Autodesk Fusion 360 part; units mm, degrees
(part 3 of 4)
  arc A110 (-253.4839, 110.4829) -> (-253.0782, 110.7207) centre (-253.4447, 110.881) ccw
  arc A111 (-251.1958, 114.9274) -> (-251.2888, 115.3883) centre (-251.5595, 115.0938) ccw
  arc A112 (-273.2935, 80.8439) -> (-274.4157, 76.9484) centre (0, 0) ccw
  spline S113 degree 3 poles (-273.2935, 80.8439) (-270.7574, 81.1159) (-268.4259, 81.2764) (-266.3051, 81.3548) knots 0 0 0 0 1 1 1 1
  spline S114 degree 3 poles (-270.6648, 56.5783) (-271.2365, 56.9046) (-271.8248, 57.2492) (-272.4294, 57.6132) knots 0 0 0 0 1 1 1 1
  arc A113 (-251.1958, 114.9274) -> (-253.0782, 110.7207) centre (0, 0) ccw
  arc A114 (-266.8977, 71.2268) -> (-267.0666, 71.6656) centre (-267.2842, 71.3299) ccw
  spline S115 degree 3 poles (-255.5218, 110.66) (-254.8182, 110.607) (-254.1389, 110.5476) (-253.4839, 110.4829) knots 0 0 0 0 1 1 1 1
  spline S116 degree 3 poles (-266.3051, 81.3548) (-265.6, 81.381) (-264.9183, 81.398) (-264.2602, 81.407) knots 0 0 0 0 1 1 1 1
  arc A115 (-246.8902, 124.5221) -> (-246.4719, 124.7367) centre (-246.8288, 124.9173) ccw
  arc A116 (-244.3566, 128.8313) -> (-246.4719, 124.7367) centre (0, 0) ccw
  arc A117 (-248.452, 139.6305) -> (-250.4129, 136.0824) centre (0, 0) ccw
  spline S117 degree 3 poles (-267.0666, 71.6656) (-267.6191, 72.0234) (-268.1872, 72.4005) (-268.7704, 72.7978) knots 0 0 0 0 1 1 1 1
  arc A118 (-274.1626, 35.9916) -> (-273.8386, 36.3324) centre (-274.2352, 36.385) ccw
  spline S118 degree 3 poles (-275.2312, 42.2473) (-277.1078, 43.2382) (-279.1389, 44.3943) (-281.3058, 45.7398) knots 0 0 0 0 1 1 1 1
  spline S119 degree 3 poles (-248.9151, 124.8131) (-248.2155, 124.7208) (-247.5406, 124.6234) (-246.8902, 124.5221) knots 0 0 0 0 1 1 1 1
  arc A119 (-273.1944, 40.8958) -> (-273.4114, 41.313) centre (-273.59, 40.9551) ccw
  spline S120 degree 3 poles (-245.8327, 130.7796) (-247.2768, 132.3347) (-248.812, 134.0968) (-250.4129, 136.0824) knots 0 0 0 0 1 1 1 1
  spline S121 degree 3 poles (-261.3246, 96.1587) (-260.6191, 96.1452) (-259.9375, 96.124) (-259.2799, 96.0962) knots 0 0 0 0 1 1 1 1
  spline S122 degree 3 poles (-251.2888, 115.3883) (-251.7735, 115.8336) (-252.2705, 116.3006) (-252.7789, 116.7899) knots 0 0 0 0 1 1 1 1
  arc A120 (-236.7485, 142.3298) -> (-239.0901, 138.3603) centre (0, 0) ccw
  arc A121 (-273.1944, 40.8958) -> (-273.8386, 36.3324) centre (0, 0) ccw
  arc A122 (-270.4716, 56.1496) -> (-270.6648, 56.5783) centre (-270.8632, 56.2309) ccw
  spline S123 degree 3 poles (-268.3306, 96.0404) (-265.7832, 96.1698) (-263.4464, 96.1992) (-261.3246, 96.1587) knots 0 0 0 0 1 1 1 1
  arc A123 (-268.409, 66.4618) -> (-268.0489, 66.7641) centre (-268.437, 66.8608) ccw
  spline S124 degree 3 poles (-257.3634, 101.1169) (-257.8723, 101.5344) (-258.3946, 101.9727) (-258.9296, 102.4328) knots 0 0 0 0 1 1 1 1
  spline S125 degree 3 poles (-268.7704, 72.7978) (-270.5243, 73.9925) (-272.4131, 75.3688) (-274.4157, 76.9484) knots 0 0 0 0 1 1 1 1
  arc A124 (-262.4841, 86.0798) -> (-262.6282, 86.5274) centre (-262.8642, 86.2044) ccw
  spline S126 degree 3 poles (-255.8902, 125.48) (-253.3445, 125.3234) (-251.019, 125.091) (-248.9151, 124.8131) knots 0 0 0 0 1 1 1 1
  arc A125 (-280.6267, 49.7364) -> (-281.3058, 45.7398) centre (0, 0) ccw
  arc A126 (-270.4716, 56.1496) -> (-271.3707, 51.6295) centre (0, 0) ccw
  arc A127 (-255.8902, 125.48) -> (-257.6492, 121.8275) centre (0, 0) ccw
  spline S127 degree 3 poles (-272.4294, 57.6132) (-274.2475, 58.7077) (-276.2105, 59.9759) (-278.2986, 61.4407) knots 0 0 0 0 1 1 1 1
  arc A128 (-262.4841, 86.0798) -> (-263.8837, 81.6887) centre (0, 0) ccw
  spline S128 degree 3 poles (-280.6267, 49.7364) (-278.137, 50.2907) (-275.8381, 50.7111) (-273.7395, 51.0266) knots 0 0 0 0 1 1 1 1
  arc A129 (-277.3965, 65.393) -> (-278.2986, 61.4407) centre (0, 0) ccw
  arc A130 (-264.2602, 81.407) -> (-263.8837, 81.6887) centre (-264.2658, 81.807) ccw
  arc A131 (-257.2447, 100.662) -> (-257.3634, 101.1169) centre (-257.6171, 100.8077) ccw
  arc A132 (-268.3306, 96.0404) -> (-269.6695, 92.214) centre (0, 0) ccw
  arc A133 (-262.5234, 110.9347) -> (-264.0748, 107.1894) centre (0, 0) ccw
  spline S129 degree 3 poles (-273.4114, 41.313) (-274.0004, 41.6067) (-274.6072, 41.9178) (-275.2312, 42.2473) knots 0 0 0 0 1 1 1 1
  spline S130 degree 3 poles (-270.4478, 66.295) (-269.7452, 66.3606) (-269.0656, 66.4158) (-268.409, 66.4618) knots 0 0 0 0 1 1 1 1
  spline S131 degree 3 poles (-252.7789, 116.7899) (-254.3079, 118.2616) (-255.9395, 119.9348) (-257.6492, 121.8275) knots 0 0 0 0 1 1 1 1
  spline S132 degree 3 poles (-264.2658, 87.7533) (-265.9499, 89.0445) (-267.7586, 90.5246) (-269.6695, 92.214) knots 0 0 0 0 1 1 1 1
  arc A134 (-271.7132, 51.3074) -> (-271.3707, 51.6295) centre (-271.7636, 51.7042) ccw
  arc A135 (-257.2447, 100.662) -> (-258.8882, 96.3563) centre (0, 0) ccw
  arc A136 (-244.3566, 128.8313) -> (-244.4236, 129.2967) centre (-244.7104, 129.0178) ccw
  spline S133 degree 3 poles (-244.4236, 129.2967) (-244.8826, 129.7685) (-245.3526, 130.2625) (-245.8327, 130.7796) knots 0 0 0 0 1 1 1 1
  spline S134 degree 3 poles (-262.6282, 86.5274) (-263.1597, 86.9156) (-263.7058, 87.324) (-264.2658, 87.7533) knots 0 0 0 0 1 1 1 1
  spline S135 degree 3 poles (-276.1699, 35.5976) (-275.4792, 35.7415) (-274.81, 35.8724) (-274.1626, 35.9916) knots 0 0 0 0 1 1 1 1
  spline S136 degree 3 poles (-273.7395, 51.0266) (-273.0417, 51.1315) (-272.3662, 51.2247) (-271.7132, 51.3074) knots 0 0 0 0 1 1 1 1
  spline S137 degree 3 poles (-258.9296, 102.4328) (-260.5388, 103.8164) (-262.2616, 105.3955) (-264.0748, 107.1894) knots 0 0 0 0 1 1 1 1
  arc A137 (-259.2799, 96.0962) -> (-258.8882, 96.3563) centre (-259.2631, 96.4958) ccw
  arc A138 (-236.7485, 142.3298) -> (-236.7894, 142.7982) centre (-237.0914, 142.5359) ccw
  spline S138 degree 3 poles (-224.4912, 164.7445) (-223.817, 164.5362) (-223.1679, 164.3272) (-222.5437, 164.1184) knots 0 0 0 0 1 1 1 1
  arc A139 (-209.5624, 179.9757) -> (-212.5358, 176.4544) centre (0, 0) ccw
  arc A140 (-211.152, 191.4154) -> (-213.8534, 188.3926) centre (0, 0) ccw
  spline S139 degree 3 poles (-248.452, 139.6305) (-245.919, 139.3314) (-243.6102, 138.969) (-241.5251, 138.5736) knots 0 0 0 0 1 1 1 1
  arc A141 (-231.3958, 151.382) -> (-230.9561, 151.5485) centre (-231.2905, 151.7679) ccw
  spline S140 degree 3 poles (-241.5251, 138.5736) (-240.8319, 138.4421) (-240.1635, 138.307) (-239.5198, 138.1694) knots 0 0 0 0 1 1 1 1
  spline S141 degree 3 poles (-219.3122, 168.4123) (-219.6856, 168.9543) (-220.0662, 169.5201) (-220.453, 170.1103) knots 0 0 0 0 1 1 1 1
  spline S142 degree 3 poles (-231.2561, 166.5703) (-228.7725, 165.9895) (-226.5188, 165.3708) (-224.4912, 164.7445) knots 0 0 0 0 1 1 1 1
  arc A142 (-222.5437, 164.1184) -> (-222.0953, 164.2599) centre (-222.4169, 164.4977) ccw
  arc A143 (-219.324, 167.9423) -> (-222.0953, 164.2599) centre (0, 0) ccw
  arc A144 (-209.5624, 179.9757) -> (-209.5242, 180.4443) centre (-209.8658, 180.2363) ccw
  spline S143 degree 3 poles (-211.152, 191.4154) (-208.7491, 190.5602) (-206.5789, 189.6931) (-204.6341, 188.8436) knots 0 0 0 0 1 1 1 1
  spline S144 degree 3 poles (-204.6341, 188.8436) (-203.9875, 188.5612) (-203.3659, 188.2808) (-202.769, 188.0034) knots 0 0 0 0 1 1 1 1
  arc A145 (-200.0871, 202.9537) -> (-202.9537, 200.0871) centre (0, 0) ccw
  spline S145 degree 3 poles (-228.4101, 155.8505) (-228.8134, 156.3707) (-229.2251, 156.9142) (-229.6443, 157.4818) knots 0 0 0 0 1 1 1 1
  spline S146 degree 3 poles (-199.077, 191.9086) (-199.3874, 192.489) (-199.7023, 193.0938) (-200.0205, 193.7236) knots 0 0 0 0 1 1 1 1
  arc A146 (-219.324, 167.9423) -> (-219.3122, 168.4123) centre (-219.6416, 168.1855) ccw
  spline S147 degree 3 poles (-200.0205, 193.7236) (-200.9776, 195.6177) (-201.965, 197.7359) (-202.9537, 200.0871) knots 0 0 0 0 1 1 1 1
  spline S148 degree 3 poles (-236.7894, 142.7982) (-237.2212, 143.295) (-237.6627, 143.8146) (-238.1131, 144.3578) knots 0 0 0 0 1 1 1 1
  spline S149 degree 3 poles (-238.1131, 144.3578) (-239.4677, 145.9914) (-240.9017, 147.8368) (-242.3888, 149.9091) knots 0 0 0 0 1 1 1 1
  spline S150 degree 3 poles (-233.3753, 151.898) (-232.6905, 151.7279) (-232.0307, 151.5555) (-231.3958, 151.382) knots 0 0 0 0 1 1 1 1
  spline S151 degree 3 poles (-214.9007, 177.0726) (-214.2393, 176.8269) (-213.6029, 176.5818) (-212.9914, 176.3383) knots 0 0 0 0 1 1 1 1
  arc A147 (-199.1414, 191.4428) -> (-199.077, 191.9086) centre (-199.4298, 191.72) ccw
  spline S152 degree 3 poles (-193.7236, 200.0205) (-193.0938, 199.7023) (-192.489, 199.3874) (-191.9086, 199.077) knots 0 0 0 0 1 1 1 1
  arc A148 (-228.3956, 155.3805) -> (-230.9561, 151.5485) centre (0, 0) ccw
  arc A149 (-221.5526, 179.2749) -> (-224.0802, 176.1054) centre (0, 0) ccw
  arc A150 (-199.1414, 191.4428) -> (-202.3076, 188.0938) centre (0, 0) ccw
  spline S153 degree 3 poles (-220.453, 170.1103) (-221.6162, 171.8853) (-222.8345, 173.8797) (-224.0802, 176.1054) knots 0 0 0 0 1 1 1 1
  arc A151 (-228.3956, 155.3805) -> (-228.4101, 155.8505) centre (-228.7263, 155.6055) ccw
  arc A152 (-212.9914, 176.3383) -> (-212.5358, 176.4544) centre (-212.8436, 176.71) ccw
  arc A153 (-202.769, 188.0034) -> (-202.3076, 188.0938) centre (-202.6005, 188.3662) ccw
  arc A154 (-188.0938, 202.3076) -> (-191.4428, 199.1414) centre (0, 0) ccw
  arc A155 (-188.0938, 202.3076) -> (-188.0034, 202.769) centre (-188.3662, 202.6005) ccw
  arc A156 (-239.5198, 138.1694) -> (-239.0901, 138.3603) centre (-239.4363, 138.5606) ccw
  arc A157 (-240.232, 153.3416) -> (-242.3888, 149.9091) centre (0, 0) ccw
  spline S154 degree 3 poles (-200.0871, 202.9537) (-197.7359, 201.965) (-195.6177, 200.9776) (-193.7236, 200.0205) knots 0 0 0 0 1 1 1 1
  spline S155 degree 3 poles (-209.5242, 180.4443) (-209.8667, 181.0064) (-210.2149, 181.5927) (-210.568, 182.2036) knots 0 0 0 0 1 1 1 1
  spline S156 degree 3 poles (-210.568, 182.2036) (-211.6298, 184.041) (-212.7344, 186.1006) (-213.8534, 188.3926) knots 0 0 0 0 1 1 1 1
  spline S157 degree 3 poles (-240.232, 153.3416) (-237.7197, 152.901) (-235.4349, 152.4097) (-233.3753, 151.898) knots 0 0 0 0 1 1 1 1
  spline S158 degree 3 poles (-229.6443, 157.4818) (-230.9052, 159.1888) (-232.2335, 161.1117) (-233.602, 163.2641) knots 0 0 0 0 1 1 1 1
  arc A158 (-231.2561, 166.5703) -> (-233.602, 163.2641) centre (0, 0) ccw
  spline S159 degree 3 poles (-221.5526, 179.2749) (-219.1055, 178.5557) (-216.89, 177.8117) (-214.9007, 177.0726) knots 0 0 0 0 1 1 1 1
  spline S160 degree 3 poles (-188.0034, 202.769) (-188.2808, 203.3659) (-188.5612, 203.9875) (-188.8436, 204.6341) knots 0 0 0 0 1 1 1 1
  arc A159 (-164.2599, 222.0953) -> (-167.9423, 219.324) centre (0, 0) ccw
  arc A160 (-155.3805, -228.3956) -> (-155.8505, -228.4101) centre (-155.6055, -228.7263) ccw
  arc A161 (-176.4544, 212.5358) -> (-179.9757, 209.5624) centre (0, 0) ccw
  arc A162 (-168.4123, 219.3122) -> (-167.9423, 219.324) centre (-168.1855, 219.6416) ccw
  spline S161 degree 3 poles (-177.0726, 214.9007) (-177.8117, 216.89) (-178.5557, 219.1055) (-179.2749, 221.5526) knots 0 0 0 0 1 1 1 1
  arc A163 (-151.5485, 230.9561) -> (-155.3805, 228.3956) centre (0, 0) ccw
  arc A164 (-155.3805, -228.3956) -> (-151.5485, -230.9561) centre (0, 0) ccw
  spline S162 degree 3 poles (-157.4818, -229.6443) (-159.1888, -230.9052) (-161.1117, -232.2335) (-163.2641, -233.602) knots 0 0 0 0 1 1 1 1
  arc A165 (-167.9423, -219.324) -> (-168.4123, -219.3122) centre (-168.1855, -219.6416) ccw
  spline S163 degree 3 poles (-168.4123, -219.3122) (-168.9543, -219.6856) (-169.5201, -220.0662) (-170.1103, -220.453) knots 0 0 0 0 1 1 1 1
  spline S164 degree 3 poles (-179.2749, -221.5526) (-178.5557, -219.1055) (-177.8117, -216.89) (-177.0726, -214.9007) knots 0 0 0 0 1 1 1 1
  spline S165 degree 3 poles (-188.8436, 204.6341) (-189.6931, 206.5789) (-190.5602, 208.7491) (-191.4154, 211.152) knots 0 0 0 0 1 1 1 1
  arc A166 (-164.2599, 222.0953) -> (-164.1184, 222.5437) centre (-164.4977, 222.4169) ccw
  spline S166 degree 3 poles (-153.3416, -240.232) (-152.901, -237.7197) (-152.4097, -235.4349) (-151.898, -233.3753) knots 0 0 0 0 1 1 1 1
  spline S167 degree 3 poles (-180.4443, -209.5242) (-181.0064, -209.8667) (-181.5927, -210.2149) (-182.2036, -210.568) knots 0 0 0 0 1 1 1 1
  arc A167 (-176.1054, 224.0802) -> (-179.2749, 221.5526) centre (0, 0) ccw
  spline S168 degree 3 poles (-151.382, 231.3958) (-151.5555, 232.0307) (-151.7279, 232.6905) (-151.898, 233.3753) knots 0 0 0 0 1 1 1 1
  arc A168 (-151.382, -231.3958) -> (-151.5485, -230.9561) centre (-151.7679, -231.2905) ccw
  arc A169 (-179.9757, -209.5624) -> (-176.4544, -212.5358) centre (0, 0) ccw
  arc A170 (-179.9757, -209.5624) -> (-180.4443, -209.5242) centre (-180.2363, -209.8658) ccw
  spline S169 degree 3 poles (-176.1054, 224.0802) (-173.8797, 222.8345) (-171.8853, 221.6162) (-170.1103, 220.453) knots 0 0 0 0 1 1 1 1
  arc A171 (-191.9086, 199.077) -> (-191.4428, 199.1414) centre (-191.72, 199.4298) ccw
  spline S170 degree 3 poles (-164.1184, 222.5437) (-164.3272, 223.1679) (-164.5362, 223.817) (-164.7445, 224.4912) knots 0 0 0 0 1 1 1 1
  spline S171 degree 3 poles (-170.1103, 220.453) (-169.5201, 220.0662) (-168.9543, 219.6856) (-168.4123, 219.3122) knots 0 0 0 0 1 1 1 1
  spline S172 degree 3 poles (-151.898, 233.3753) (-152.4097, 235.4349) (-152.901, 237.7197) (-153.3416, 240.232) knots 0 0 0 0 1 1 1 1
  arc A172 (-155.8505, 228.4101) -> (-155.3805, 228.3956) centre (-155.6055, 228.7263) ccw
  arc A173 (-188.3926, 213.8534) -> (-191.4154, 211.152) centre (0, 0) ccw
  spline S173 degree 3 poles (-188.3926, 213.8534) (-186.1006, 212.7344) (-184.041, 211.6298) (-182.2036, 210.568) knots 0 0 0 0 1 1 1 1
  arc A174 (-149.9091, 242.3888) -> (-153.3416, 240.232) centre (0, 0) ccw
  spline S174 degree 3 poles (-151.898, -233.3753) (-151.7279, -232.6905) (-151.5555, -232.0307) (-151.382, -231.3958) knots 0 0 0 0 1 1 1 1
  spline S175 degree 3 poles (-164.7445, -224.4912) (-164.5362, -223.817) (-164.3272, -223.1679) (-164.1184, -222.5437) knots 0 0 0 0 1 1 1 1
  spline S176 degree 3 poles (-155.8505, -228.4101) (-156.3707, -228.8134) (-156.9142, -229.2251) (-157.4818, -229.6443) knots 0 0 0 0 1 1 1 1
  spline S177 degree 3 poles (-191.4154, -211.152) (-190.5602, -208.7491) (-189.6931, -206.5789) (-188.8436, -204.6341) knots 0 0 0 0 1 1 1 1
  spline S178 degree 3 poles (-177.0726, -214.9007) (-176.8269, -214.2393) (-176.5818, -213.6029) (-176.3383, -212.9914) knots 0 0 0 0 1 1 1 1
  arc A175 (-180.4443, 209.5242) -> (-179.9757, 209.5624) centre (-180.2363, 209.8658) ccw
  spline S179 degree 3 poles (-182.2036, -210.568) (-184.041, -211.6298) (-186.1006, -212.7344) (-188.3926, -213.8534) knots 0 0 0 0 1 1 1 1
  spline S180 degree 3 poles (-182.2036, 210.568) (-181.5927, 210.2149) (-181.0064, 209.8667) (-180.4443, 209.5242) knots 0 0 0 0 1 1 1 1
  arc A176 (-164.1184, -222.5437) -> (-164.2599, -222.0953) centre (-164.4977, -222.4169) ccw
  spline S181 degree 3 poles (-176.3383, 212.9914) (-176.5818, 213.6029) (-176.8269, 214.2393) (-177.0726, 214.9007) knots 0 0 0 0 1 1 1 1
  arc A177 (-151.5485, 230.9561) -> (-151.382, 231.3958) centre (-151.7679, 231.2905) ccw
  arc A178 (-166.5703, -231.2561) -> (-163.2641, -233.602) centre (0, 0) ccw
  spline S182 degree 3 poles (-170.1103, -220.453) (-171.8853, -221.6162) (-173.8797, -222.8345) (-176.1054, -224.0802) knots 0 0 0 0 1 1 1 1
  arc A179 (-179.2749, -221.5526) -> (-176.1054, -224.0802) centre (0, 0) ccw
  arc A180 (-176.3383, -212.9914) -> (-176.4544, -212.5358) centre (-176.71, -212.8436) ccw
  arc A181 (-163.2641, 233.602) -> (-166.5703, 231.2561) centre (0, 0) ccw
  arc A182 (-191.4154, -211.152) -> (-188.3926, -213.8534) centre (0, 0) ccw
  spline S183 degree 3 poles (-188.8436, -204.6341) (-188.5612, -203.9875) (-188.2808, -203.3659) (-188.0034, -202.769) knots 0 0 0 0 1 1 1 1
  spline S184 degree 3 poles (-166.5703, -231.2561) (-165.9895, -228.7725) (-165.3708, -226.5188) (-164.7445, -224.4912) knots 0 0 0 0 1 1 1 1
  arc A183 (-191.4428, -199.1414) -> (-188.0938, -202.3076) centre (0, 0) ccw
  arc A184 (-191.4428, -199.1414) -> (-191.9086, -199.077) centre (-191.72, -199.4298) ccw
  spline S185 degree 3 poles (-191.9086, -199.077) (-192.489, -199.3874) (-193.0938, -199.7023) (-193.7236, -200.0205) knots 0 0 0 0 1 1 1 1
  spline S186 degree 3 poles (-193.7236, -200.0205) (-195.6177, -200.9776) (-197.7359, -201.965) (-200.0871, -202.9537) knots 0 0 0 0 1 1 1 1
  spline S187 degree 3 poles (-157.4818, 229.6443) (-156.9142, 229.2251) (-156.3707, 228.8134) (-155.8505, 228.4101) knots 0 0 0 0 1 1 1 1
  arc A185 (-167.9423, -219.324) -> (-164.2599, -222.0953) centre (0, 0) ccw
  arc A186 (-188.0034, -202.769) -> (-188.0938, -202.3076) centre (-188.3662, -202.6005) ccw
  arc A187 (-202.9537, -200.0871) -> (-200.0871, -202.9537) centre (0, 0) ccw
  arc A188 (-176.4544, 212.5358) -> (-176.3383, 212.9914) centre (-176.71, 212.8436) ccw
  spline S188 degree 3 poles (-164.7445, 224.4912) (-165.3708, 226.5188) (-165.9895, 228.7725) (-166.5703, 231.2561) knots 0 0 0 0 1 1 1 1
  spline S189 degree 3 poles (-163.2641, 233.602) (-161.1117, 232.2335) (-159.1888, 230.9052) (-157.4818, 229.6443) knots 0 0 0 0 1 1 1 1
  spline S190 degree 3 poles (-224.4912, -164.7445) (-226.5188, -165.3708) (-228.7725, -165.9895) (-231.2561, -166.5703) knots 0 0 0 0 1 1 1 1
  spline S191 degree 3 poles (-204.6341, -188.8436) (-206.5789, -189.6931) (-208.7491, -190.5602) (-211.152, -191.4154) knots 0 0 0 0 1 1 1 1
  spline S192 degree 3 poles (-214.9007, -177.0726) (-216.89, -177.8117) (-219.1055, -178.5557) (-221.5526, -179.2749) knots 0 0 0 0 1 1 1 1
  arc A189 (-239.0901, -138.3603) -> (-236.7485, -142.3298) centre (0, 0) ccw
  arc A190 (-242.3888, -149.9091) -> (-240.232, -153.3416) centre (0, 0) ccw
  arc A191 (-222.0953, -164.2599) -> (-219.324, -167.9423) centre (0, 0) ccw
  arc A192 (-222.0953, -164.2599) -> (-222.5437, -164.1184) centre (-222.4169, -164.4977) ccw
  arc A193 (-199.077, -191.9086) -> (-199.1414, -191.4428) centre (-199.4298, -191.72) ccw
  arc A194 (-212.5358, -176.4544) -> (-209.5624, -179.9757) centre (0, 0) ccw
  arc A195 (-212.5358, -176.4544) -> (-212.9914, -176.3383) centre (-212.8436, -176.71) ccw
  spline S193 degree 3 poles (-212.9914, -176.3383) (-213.6029, -176.5818) (-214.2393, -176.8269) (-214.9007, -177.0726) knots 0 0 0 0 1 1 1 1
  arc A196 (-236.7894, -142.7982) -> (-236.7485, -142.3298) centre (-237.0914, -142.5359) ccw
  arc A197 (-246.4719, -124.7367) -> (-244.3566, -128.8313) centre (0, 0) ccw
  spline S194 degree 3 poles (-224.0802, -176.1054) (-222.8345, -173.8797) (-221.6162, -171.8853) (-220.453, -170.1103) knots 0 0 0 0 1 1 1 1
  spline S195 degree 3 poles (-231.3958, -151.382) (-232.0307, -151.5555) (-232.6905, -151.7279) (-233.3753, -151.898) knots 0 0 0 0 1 1 1 1
  spline S196 degree 3 poles (-238.1131, -144.3578) (-237.6627, -143.8146) (-237.2212, -143.295) (-236.7894, -142.7982) knots 0 0 0 0 1 1 1 1
  arc A198 (-219.3122, -168.4123) -> (-219.324, -167.9423) centre (-219.6416, -168.1855) ccw
  spline S197 degree 3 poles (-220.453, -170.1103) (-220.0662, -169.5201) (-219.6856, -168.9543) (-219.3122, -168.4123) knots 0 0 0 0 1 1 1 1
  spline S198 degree 3 poles (-200.0205, -193.7236) (-199.7023, -193.0938) (-199.3874, -192.489) (-199.077, -191.9086) knots 0 0 0 0 1 1 1 1
  arc A199 (-233.602, -163.2641) -> (-231.2561, -166.5703) centre (0, 0) ccw
  spline S199 degree 3 poles (-222.5437, -164.1184) (-223.1679, -164.3272) (-223.817, -164.5362) (-224.4912, -164.7445) knots 0 0 0 0 1 1 1 1
  arc A200 (-209.5242, -180.4443) -> (-209.5624, -179.9757) centre (-209.8658, -180.2363) ccw
  arc A201 (-228.4101, -155.8505) -> (-228.3956, -155.3805) centre (-228.7263, -155.6055) ccw
  spline S200 degree 3 poles (-229.6443, -157.4818) (-229.2251, -156.9142) (-228.8134, -156.3707) (-228.4101, -155.8505) knots 0 0 0 0 1 1 1 1
  arc A202 (-213.8534, -188.3926) -> (-211.152, -191.4154) centre (0, 0) ccw
  arc A203 (-239.0901, -138.3603) -> (-239.5198, -138.1694) centre (-239.4363, -138.5606) ccw
  spline S201 degree 3 poles (-241.5251, -138.5736) (-243.6102, -138.969) (-245.919, -139.3314) (-248.452, -139.6305) knots 0 0 0 0 1 1 1 1
  spline S202 degree 3 poles (-245.8327, -130.7796) (-245.3526, -130.2625) (-244.8826, -129.7685) (-244.4236, -129.2967) knots 0 0 0 0 1 1 1 1
  arc A204 (-246.4719, -124.7367) -> (-246.8902, -124.5221) centre (-246.8288, -124.9173) ccw
  arc A205 (-202.3076, -188.0938) -> (-199.1414, -191.4428) centre (0, 0) ccw
  arc A206 (-202.3076, -188.0938) -> (-202.769, -188.0034) centre (-202.6005, -188.3662) ccw
  spline S203 degree 3 poles (-202.9537, -200.0871) (-201.965, -197.7359) (-200.9776, -195.6177) (-200.0205, -193.7236) knots 0 0 0 0 1 1 1 1
  spline S204 degree 3 poles (-233.602, -163.2641) (-232.2335, -161.1117) (-230.9052, -159.1888) (-229.6443, -157.4818) knots 0 0 0 0 1 1 1 1
  arc A207 (-230.9561, -151.5485) -> (-228.3956, -155.3805) centre (0, 0) ccw
  arc A208 (-230.9561, -151.5485) -> (-231.3958, -151.382) centre (-231.2905, -151.7679) ccw
  spline S205 degree 3 poles (-239.5198, -138.1694) (-240.1635, -138.307) (-240.8319, -138.4421) (-241.5251, -138.5736) knots 0 0 0 0 1 1 1 1
  arc A209 (-244.4236, -129.2967) -> (-244.3566, -128.8313) centre (-244.7104, -129.0178) ccw
  spline S206 degree 3 poles (-246.8902, -124.5221) (-247.5406, -124.6234) (-248.2155, -124.7208) (-248.9151, -124.8131) knots 0 0 0 0 1 1 1 1
  spline S207 degree 3 poles (-202.769, -188.0034) (-203.3659, -188.2808) (-203.9875, -188.5612) (-204.6341, -188.8436) knots 0 0 0 0 1 1 1 1
  spline S208 degree 3 poles (-248.9151, -124.8131) (-251.019, -125.091) (-253.3445, -125.3234) (-255.8902, -125.48) knots 0 0 0 0 1 1 1 1
  arc A210 (-224.0802, -176.1054) -> (-221.5526, -179.2749) centre (0, 0) ccw
  arc A211 (-257.6492, -121.8275) -> (-255.8902, -125.48) centre (0, 0) ccw
  spline S209 degree 3 poles (-213.8534, -188.3926) (-212.7344, -186.1006) (-211.6298, -184.041) (-210.568, -182.2036) knots 0 0 0 0 1 1 1 1
  spline S210 degree 3 poles (-210.568, -182.2036) (-210.2149, -181.5927) (-209.8667, -181.0064) (-209.5242, -180.4443) knots 0 0 0 0 1 1 1 1
  spline S211 degree 3 poles (-250.4129, -136.0824) (-248.812, -134.0968) (-247.2768, -132.3347) (-245.8327, -130.7796) knots 0 0 0 0 1 1 1 1
  spline S212 degree 3 poles (-242.3888, -149.9091) (-240.9017, -147.8368) (-239.4677, -145.9914) (-238.1131, -144.3578) knots 0 0 0 0 1 1 1 1
  arc A212 (-250.4129, -136.0824) -> (-248.452, -139.6305) centre (0, 0) ccw
  spline S213 degree 3 poles (-233.3753, -151.898) (-235.4349, -152.4097) (-237.7197, -152.901) (-240.232, -153.3416) knots 0 0 0 0 1 1 1 1
  spline S214 degree 3 poles (-266.3051, -81.3548) (-268.4259, -81.2764) (-270.7574, -81.1159) (-273.2935, -80.8439) knots 0 0 0 0 1 1 1 1
  spline S215 degree 3 poles (-274.4157, -76.9484) (-272.4131, -75.3688) (-270.5243, -73.9925) (-268.7704, -72.7978) knots 0 0 0 0 1 1 1 1
  spline S216 degree 3 poles (-271.7132, -51.3074) (-272.3662, -51.2247) (-273.0417, -51.1315) (-273.7395, -51.0266) knots 0 0 0 0 1 1 1 1
  spline S217 degree 3 poles (-259.2799, -96.0962) (-259.9375, -96.124) (-260.6191, -96.1452) (-261.3246, -96.1587) knots 0 0 0 0 1 1 1 1
  spline S218 degree 3 poles (-268.409, -66.4618) (-269.0656, -66.4158) (-269.7452, -66.3606) (-270.4478, -66.295) knots 0 0 0 0 1 1 1 1
  arc A213 (-268.0489, -66.7641) -> (-268.409, -66.4618) centre (-268.437, -66.8608) ccw
  spline S219 degree 3 poles (-257.6492, -121.8275) (-255.9395, -119.9348) (-254.3079, -118.2616) (-252.7789, -116.7899) knots 0 0 0 0 1 1 1 1
  spline S220 degree 3 poles (-264.0748, -107.1894) (-262.2616, -105.3955) (-260.5388, -103.8164) (-258.9296, -102.4328) knots 0 0 0 0 1 1 1 1
  spline S221 degree 3 poles (-281.3058, -45.7398) (-279.1389, -44.3943) (-277.1078, -43.2382) (-275.2312, -42.2473) knots 0 0 0 0 1 1 1 1
  arc A214 (-262.6282, -86.5274) -> (-262.4841, -86.0798) centre (-262.8642, -86.2044) ccw
  spline S222 degree 3 poles (-278.2986, -61.4407) (-276.2105, -59.9759) (-274.2475, -58.7077) (-272.4294, -57.6132) knots 0 0 0 0 1 1 1 1
  arc A215 (-273.8386, -36.3324) -> (-273.1944, -40.8958) centre (0, 0) ccw
  spline S223 degree 3 poles (-274.1626, -35.9916) (-274.81, -35.8724) (-275.4792, -35.7415) (-276.1699, -35.5976) knots 0 0 0 0 1 1 1 1
  spline S224 degree 3 poles (-275.2312, -42.2473) (-274.6072, -41.9178) (-274.0004, -41.6067) (-273.4114, -41.313) knots 0 0 0 0 1 1 1 1
  arc A216 (-273.8386, -36.3324) -> (-274.1626, -35.9916) centre (-274.2352, -36.385) ccw
  spline S225 degree 3 poles (-261.3246, -96.1587) (-263.4464, -96.1992) (-265.7832, -96.1698) (-268.3306, -96.0404) knots 0 0 0 0 1 1 1 1
  spline S226 degree 3 poles (-276.1699, -35.5976) (-278.2476, -35.165) (-280.5193, -34.6163) (-282.974, -33.9233) knots 0 0 0 0 1 1 1 1
  spline S227 degree 3 poles (-283.4279, -29.8949) (-281.1889, -28.673) (-279.0963, -27.6326) (-277.167, -26.7485) knots 0 0 0 0 1 1 1 1
  arc A217 (-278.2986, -61.4407) -> (-277.3965, -65.393) centre (0, 0) ccw
  arc A218 (-273.4114, -41.313) -> (-273.1944, -40.8958) centre (-273.59, -40.9551) ccw
  arc A219 (-268.0489, -66.7641) -> (-266.8977, -71.2268) centre (0, 0) ccw
  arc A220 (-251.2888, -115.3883) -> (-251.1958, -114.9274) centre (-251.5595, -115.0938) ccw
  arc A221 (-264.0748, -107.1894) -> (-262.5234, -110.9347) centre (0, 0) ccw
  spline S228 degree 3 poles (-255.5218, -110.66) (-257.638, -110.8195) (-259.9728, -110.9211) (-262.5234, -110.9347) knots 0 0 0 0 1 1 1 1
  arc A222 (-258.8882, -96.3563) -> (-257.2447, -100.662) centre (0, 0) ccw
  arc A223 (-258.8882, -96.3563) -> (-259.2799, -96.0962) centre (-259.2631, -96.4958) ccw
  arc A224 (-267.0666, -71.6656) -> (-266.8977, -71.2268) centre (-267.2842, -71.3299) ccw
  spline S229 degree 3 poles (-273.7395, -51.0266) (-275.8381, -50.7111) (-278.137, -50.2907) (-280.6267, -49.7364) knots 0 0 0 0 1 1 1 1
  arc A225 (-257.3634, -101.1169) -> (-257.2447, -100.662) centre (-257.6171, -100.8077) ccw
  arc A226 (-253.0782, -110.7207) -> (-253.4839, -110.4829) centre (-253.4447, -110.881) ccw
  spline S230 degree 3 poles (-253.4839, -110.4829) (-254.1389, -110.5476) (-254.8182, -110.607) (-255.5218, -110.66) knots 0 0 0 0 1 1 1 1
  arc A227 (-269.6695, -92.214) -> (-268.3306, -96.0404) centre (0, 0) ccw
  arc A228 (-274.4157, -76.9484) -> (-273.2935, -80.8439) centre (0, 0) ccw
  spline S231 degree 3 poles (-252.7789, -116.7899) (-252.2705, -116.3006) (-251.7735, -115.8336) (-251.2888, -115.3883) knots 0 0 0 0 1 1 1 1
  spline S232 degree 3 poles (-264.2602, -81.407) (-264.9183, -81.398) (-265.6, -81.381) (-266.3051, -81.3548) knots 0 0 0 0 1 1 1 1
  spline S233 degree 3 poles (-268.7704, -72.7978) (-268.1872, -72.4005) (-267.6191, -72.0234) (-267.0666, -71.6656) knots 0 0 0 0 1 1 1 1
  arc A229 (-253.0782, -110.7207) -> (-251.1958, -114.9274) centre (0, 0) ccw
  arc A230 (-263.8837, -81.6887) -> (-264.2602, -81.407) centre (-264.2658, -81.807) ccw
  spline S234 degree 3 poles (-264.2658, -87.7533) (-263.7058, -87.324) (-263.1597, -86.9156) (-262.6282, -86.5274) knots 0 0 0 0 1 1 1 1
  arc A231 (-271.3707, -51.6295) -> (-270.4716, -56.1496) centre (0, 0) ccw
  arc A232 (-271.3707, -51.6295) -> (-271.7132, -51.3074) centre (-271.7636, -51.7042) ccw
  arc A233 (-263.8837, -81.6887) -> (-262.4841, -86.0798) centre (0, 0) ccw
  arc A234 (-270.6648, -56.5783) -> (-270.4716, -56.1496) centre (-270.8632, -56.2309) ccw
  spline S235 degree 3 poles (-272.4294, -57.6132) (-271.8248, -57.2492) (-271.2365, -56.9046) (-270.6648, -56.5783) knots 0 0 0 0 1 1 1 1
  spline S236 degree 3 poles (-258.9296, -102.4328) (-258.3946, -101.9727) (-257.8723, -101.5344) (-257.3634, -101.1169) knots 0 0 0 0 1 1 1 1
  arc A235 (-281.3058, -45.7398) -> (-280.6267, -49.7364) centre (0, 0) ccw
  spline S237 degree 3 poles (-269.6695, -92.214) (-267.7586, -90.5246) (-265.9499, -89.0445) (-264.2658, -87.7533) knots 0 0 0 0 1 1 1 1
  spline S238 degree 3 poles (-270.4478, -66.295) (-272.5608, -66.0977) (-274.8797, -65.8068) (-277.3965, -65.393) knots 0 0 0 0 1 1 1 1
  spline S239 degree 3 poles (-275.7494, -20.5626) (-276.389, -20.4073) (-277.0498, -20.239) (-277.7315, -20.0566) knots 0 0 0 0 1 1 1 1
  spline S240 degree 3 poles (-142.7982, -236.7894) (-143.295, -237.2212) (-143.8146, -237.6627) (-144.3578, -238.1131) knots 0 0 0 0 1 1 1 1
  spline S241 degree 3 poles (51.3074, -271.7132) (51.2247, -272.3662) (51.1315, -273.0417) (51.0266, -273.7395) knots 0 0 0 0 1 1 1 1
  spline S242 degree 3 poles (-278.2308, -11.1655) (-277.5738, -10.908) (-276.936, -10.6668) (-276.3178, -10.4408) knots 0 0 0 0 1 1 1 1
  arc A236 (-142.3298, -236.7485) -> (-142.7982, -236.7894) centre (-142.5359, -237.0914) ccw
  spline S243 degree 3 poles (-144.3578, -238.1131) (-145.9914, -239.4677) (-147.8368, -240.9017) (-149.9091, -242.3888) knots 0 0 0 0 1 1 1 1
  spline S244 degree 3 poles (57.6132, -272.4294) (57.2492, -271.8248) (56.9046, -271.2365) (56.5783, -270.6648) knots 0 0 0 0 1 1 1 1
  arc A237 (51.6295, -271.3707) -> (56.1496, -270.4716) centre (0, 0) ccw
  arc A238 (-275.2977, -25.9177) -> (-275.0576, -25.5134) centre (-275.4559, -25.5503) ccw
  spline S245 degree 3 poles (-138.5736, -241.5251) (-138.4421, -240.8319) (-138.307, -240.1635) (-138.1694, -239.5198) knots 0 0 0 0 1 1 1 1
  arc A239 (-275.445, -20.921) -> (-275.7494, -20.5626) centre (-275.8439, -20.9513) ccw
  spline S246 degree 3 poles (42.2473, -275.2312) (41.9178, -274.6072) (41.6067, -274.0004) (41.313, -273.4114) knots 0 0 0 0 1 1 1 1
  arc A240 (51.6295, -271.3707) -> (51.3074, -271.7132) centre (51.7042, -271.7636) ccw
  arc A241 (41.313, -273.4114) -> (40.8958, -273.1944) centre (40.9551, -273.59) ccw
  arc A242 (45.7398, -281.3058) -> (49.7364, -280.6267) centre (0, 0) ccw
  arc A243 (29.8949, -283.4279) -> (33.9233, -282.974) centre (0, 0) ccw
  arc A244 (-139.6305, -248.452) -> (-136.0824, -250.4129) centre (0, 0) ccw
  spline S247 degree 3 poles (-277.167, -26.7485) (-276.5255, -26.4545) (-275.9023, -26.1779) (-275.2977, -25.9177) knots 0 0 0 0 1 1 1 1
  arc A245 (36.3324, -273.8386) -> (35.9916, -274.1626) centre (36.385, -274.2352) ccw
  spline S248 degree 3 poles (-284.6582, -13.9559) (-282.3543, -12.8615) (-280.2066, -11.94) (-278.2308, -11.1655) knots 0 0 0 0 1 1 1 1
  arc A246 (-275.445, -20.921) -> (-275.0576, -25.5134) centre (0, 0) ccw
  arc A247 (-276.1847, -5.4437) -> (-276.0555, -10.0506) centre (0, 0) ccw
  arc A248 (-142.3298, -236.7485) -> (-138.3603, -239.0901) centre (0, 0) ccw
  arc A249 (-138.1694, -239.5198) -> (-138.3603, -239.0901) centre (-138.5606, -239.4363) ccw
  spline S249 degree 3 poles (35.5976, -276.1699) (35.165, -278.2476) (34.6163, -280.5193) (33.9233, -282.974) knots 0 0 0 0 1 1 1 1
  spline S250 degree 3 poles (29.8949, -283.4279) (28.673, -281.1889) (27.6326, -279.0963) (26.7485, -277.167) knots 0 0 0 0 1 1 1 1
  arc A250 (25.9177, -275.2977) -> (25.5134, -275.0576) centre (25.5503, -275.4559) ccw
  arc A251 (20.921, -275.445) -> (20.5626, -275.7494) centre (20.9513, -275.8439) ccw
  arc A252 (20.921, -275.445) -> (25.5134, -275.0576) centre (0, 0) ccw
  spline S251 degree 3 poles (-277.7315, -20.0566) (-279.7816, -19.5082) (-282.0189, -18.833) (-284.4309, -18.0035) knots 0 0 0 0 1 1 1 1
  arc A253 (-276.3178, -10.4408) -> (-276.0555, -10.0506) centre (-276.4552, -10.0652) ccw
  spline S252 degree 3 poles (20.5626, -275.7494) (20.4073, -276.389) (20.239, -277.0498) (20.0566, -277.7315) knots 0 0 0 0 1 1 1 1
  arc A254 (-153.3416, -240.232) -> (-149.9091, -242.3888) centre (0, 0) ccw
  spline S253 degree 3 poles (35.9916, -274.1626) (35.8724, -274.81) (35.7415, -275.4792) (35.5976, -276.1699) knots 0 0 0 0 1 1 1 1
  spline S254 degree 3 poles (20.0566, -277.7315) (19.5082, -279.7816) (18.833, -282.0189) (18.0035, -284.4309) knots 0 0 0 0 1 1 1 1
  arc A255 (13.9559, -284.6582) -> (18.0035, -284.4309) centre (0, 0) ccw
  arc A256 (5.4437, -276.1847) -> (10.0506, -276.0555) centre (0, 0) ccw
  spline S255 degree 3 poles (-129.2967, -244.4236) (-129.7685, -244.8826) (-130.2625, -245.3526) (-130.7796, -245.8327) knots 0 0 0 0 1 1 1 1
  arc A257 (-283.4279, -29.8949) -> (-282.974, -33.9233) centre (0, 0) ccw
  arc A258 (-284.6582, -13.9559) -> (-284.4309, -18.0035) centre (0, 0) ccw
  spline S256 degree 3 poles (-139.6305, -248.452) (-139.3314, -245.919) (-138.969, -243.6102) (-138.5736, -241.5251) knots 0 0 0 0 1 1 1 1
  arc A259 (56.5783, -270.6648) -> (56.1496, -270.4716) centre (56.2309, -270.8632) ccw
  spline S257 degree 3 poles (45.7398, -281.3058) (44.3943, -279.1389) (43.2382, -277.1078) (42.2473, -275.2312) knots 0 0 0 0 1 1 1 1
  arc A260 (36.3324, -273.8386) -> (40.8958, -273.1944) centre (0, 0) ccw
  spline S258 degree 3 poles (26.7485, -277.167) (26.4545, -276.5255) (26.1779, -275.9023) (25.9177, -275.2977) knots 0 0 0 0 1 1 1 1
  spline S259 degree 3 poles (51.0266, -273.7395) (50.7111, -275.8381) (50.2907, -278.137) (49.7364, -280.6267) knots 0 0 0 0 1 1 1 1
  arc A261 (-276.1847, -5.4437) -> (-276.4685, -5.0688) centre (-276.5847, -5.4516) ccw
  spline S260 degree 3 poles (-130.7796, -245.8327) (-132.3347, -247.2768) (-134.0968, -248.812) (-136.0824, -250.4129) knots 0 0 0 0 1 1 1 1
  arc A262 (-2.027, -284.9929) -> (2.027, -284.9929) centre (0, 0) ccw
  spline S261 degree 3 poles (-18.0035, -284.4309) (-18.833, -282.0189) (-19.5082, -279.7816) (-20.0566, -277.7315) knots 0 0 0 0 1 1 1 1
  spline S262 degree 3 poles (-49.7364, -280.6267) (-50.2907, -278.137) (-50.7111, -275.8381) (-51.0266, -273.7395) knots 0 0 0 0 1 1 1 1
  arc A263 (-56.1496, -270.4716) -> (-51.6295, -271.3707) centre (0, 0) ccw
  arc A264 (10.4408, -276.3178) -> (10.0506, -276.0555) centre (10.0652, -276.4552) ccw
  spline S263 degree 3 poles (-10.4408, -276.3178) (-10.6668, -276.936) (-10.908, -277.5738) (-11.1655, -278.2308) knots 0 0 0 0 1 1 1 1
  arc A265 (-18.0035, -284.4309) -> (-13.9559, -284.6582) centre (0, 0) ccw
  arc A266 (-25.5134, -275.0576) -> (-20.921, -275.445) centre (0, 0) ccw
  arc A267 (-20.5626, -275.7494) -> (-20.921, -275.445) centre (-20.9513, -275.8439) ccw
  spline S264 degree 3 poles (-20.0566, -277.7315) (-20.239, -277.0498) (-20.4073, -276.389) (-20.5626, -275.7494) knots 0 0 0 0 1 1 1 1
  spline S265 degree 3 poles (-42.2473, -275.2312) (-43.2382, -277.1078) (-44.3943, -279.1389) (-45.7398, -281.3058) knots 0 0 0 0 1 1 1 1
  spline S266 degree 3 poles (-57.6132, -272.4294) (-58.7077, -274.2475) (-59.9759, -276.2105) (-61.4407, -278.2986) knots 0 0 0 0 1 1 1 1
  arc A268 (-10.0506, -276.0555) -> (-5.4437, -276.1847) centre (0, 0) ccw
  arc A269 (-40.8958, -273.1944) -> (-36.3324, -273.8386) centre (0, 0) ccw
  arc A270 (-65.393, -277.3965) -> (-61.4407, -278.2986) centre (0, 0) ccw
  arc A271 (-66.4618, -268.409) -> (-66.7641, -268.0489) centre (-66.8608, -268.437) ccw
  arc A272 (-71.2268, -266.8977) -> (-66.7641, -268.0489) centre (0, 0) ccw
  spline S267 degree 3 poles (-80.8439, -273.2935) (-81.1159, -270.7574) (-81.2764, -268.4259) (-81.3548, -266.3051) knots 0 0 0 0 1 1 1 1
  spline S268 degree 3 poles (-71.6656, -267.0666) (-72.0234, -267.6191) (-72.4005, -268.1872) (-72.7978, -268.7704) knots 0 0 0 0 1 1 1 1
  spline S269 degree 3 poles (-86.5274, -262.6282) (-86.9156, -263.1597) (-87.324, -263.7058) (-87.7533, -264.2658) knots 0 0 0 0 1 1 1 1
  spline S270 degree 3 poles (-33.9233, -282.974) (-34.6163, -280.5193) (-35.165, -278.2476) (-35.5976, -276.1699) knots 0 0 0 0 1 1 1 1
  arc A273 (-49.7364, -280.6267) -> (-45.7398, -281.3058) centre (0, 0) ccw
  spline S271 degree 3 poles (-81.3548, -266.3051) (-81.381, -265.6) (-81.398, -264.9183) (-81.407, -264.2602) knots 0 0 0 0 1 1 1 1
  arc A274 (-10.0506, -276.0555) -> (-10.4408, -276.3178) centre (-10.0652, -276.4552) ccw
  spline S272 degree 3 poles (-4.4526, -278.4191) (-4.6729, -277.7488) (-4.8779, -277.0984) (-5.0688, -276.4685) knots 0 0 0 0 1 1 1 1
  spline S273 degree 3 poles (-65.393, -277.3965) (-65.8068, -274.8797) (-66.0977, -272.5608) (-66.295, -270.4478) knots 0 0 0 0 1 1 1 1
  spline S274 degree 3 poles (-96.0404, -268.3306) (-96.1698, -265.7832) (-96.1992, -263.4464) (-96.1587, -261.3246) knots 0 0 0 0 1 1 1 1
  spline S275 degree 3 poles (4.4526, -278.4191) (3.79, -280.4352) (2.9904, -282.6312) (2.027, -284.9929) knots 0 0 0 0 1 1 1 1
  spline S276 degree 3 poles (-66.295, -270.4478) (-66.3606, -269.7452) (-66.4158, -269.0656) (-66.4618, -268.409) knots 0 0 0 0 1 1 1 1
  spline S277 degree 3 poles (-11.1655, -278.2308) (-11.94, -280.2066) (-12.8615, -282.3543) (-13.9559, -284.6582) knots 0 0 0 0 1 1 1 1
  spline S278 degree 3 poles (-35.5976, -276.1699) (-35.7415, -275.4792) (-35.8724, -274.81) (-35.9916, -274.1626) knots 0 0 0 0 1 1 1 1
  arc A275 (-86.0798, -262.4841) -> (-81.6887, -263.8837) centre (0, 0) ccw
  spline S279 degree 3 poles (-87.7533, -264.2658) (-89.0445, -265.9499) (-90.5246, -267.7586) (-92.214, -269.6695) knots 0 0 0 0 1 1 1 1
  arc A276 (-96.0404, -268.3306) -> (-92.214, -269.6695) centre (0, 0) ccw
  arc A277 (-86.0798, -262.4841) -> (-86.5274, -262.6282) centre (-86.2044, -262.8642) ccw
  spline S280 degree 3 poles (-101.1169, -257.3634) (-101.5344, -257.8723) (-101.9727, -258.3946) (-102.4328, -258.9296) knots 0 0 0 0 1 1 1 1
  arc A278 (-56.1496, -270.4716) -> (-56.5783, -270.6648) centre (-56.2309, -270.8632) ccw
  arc A279 (-40.8958, -273.1944) -> (-41.313, -273.4114) centre (-40.9551, -273.59) ccw
  arc A280 (-80.8439, -273.2935) -> (-76.9484, -274.4157) centre (0, 0) ccw
  arc A281 (-51.3074, -271.7132) -> (-51.6295, -271.3707) centre (-51.7042, -271.7636) ccw
  spline S281 degree 3 poles (5.0688, -276.4685) (4.8779, -277.0984) (4.6729, -277.7488) (4.4526, -278.4191) knots 0 0 0 0 1 1 1 1
  spline S282 degree 3 poles (-26.7485, -277.167) (-27.6326, -279.0963) (-28.673, -281.1889) (-29.8949, -283.4279) knots 0 0 0 0 1 1 1 1
  arc A282 (-81.407, -264.2602) -> (-81.6887, -263.8837) centre (-81.807, -264.2658) ccw
  arc A283 (-25.5134, -275.0576) -> (-25.9177, -275.2977) centre (-25.5503, -275.4559) ccw
  spline S283 degree 3 poles (-2.027, -284.9929) (-2.9904, -282.6312) (-3.79, -280.4352) (-4.4526, -278.4191) knots 0 0 0 0 1 1 1 1
  spline S284 degree 3 poles (11.1655, -278.2308) (10.908, -277.5738) (10.6668, -276.936) (10.4408, -276.3178) knots 0 0 0 0 1 1 1 1
  spline S285 degree 3 poles (-51.0266, -273.7395) (-51.1315, -273.0417) (-51.2247, -272.3662) (-51.3074, -271.7132) knots 0 0 0 0 1 1 1 1
  spline S286 degree 3 poles (-72.7978, -268.7704) (-73.9925, -270.5243) (-75.3688, -272.4131) (-76.9484, -274.4157) knots 0 0 0 0 1 1 1 1
  arc A284 (-100.662, -257.2447) -> (-96.3563, -258.8882) centre (0, 0) ccw
  arc A285 (-35.9916, -274.1626) -> (-36.3324, -273.8386) centre (-36.385, -274.2352) ccw
  arc A286 (-33.9233, -282.974) -> (-29.8949, -283.4279) centre (0, 0) ccw
  spline S287 degree 3 poles (-96.1587, -261.3246) (-96.1452, -260.6191) (-96.124, -259.9375) (-96.0962, -259.2799) knots 0 0 0 0 1 1 1 1
  arc A287 (-71.2268, -266.8977) -> (-71.6656, -267.0666) centre (-71.3299, -267.2842) ccw
  arc A288 (5.4437, -276.1847) -> (5.0688, -276.4685) centre (5.4516, -276.5847) ccw
  spline S288 degree 3 poles (-25.9177, -275.2977) (-26.1779, -275.9023) (-26.4545, -276.5255) (-26.7485, -277.167) knots 0 0 0 0 1 1 1 1
  spline S289 degree 3 poles (-56.5783, -270.6648) (-56.9046, -271.2365) (-57.2492, -271.8248) (-57.6132, -272.4294) knots 0 0 0 0 1 1 1 1
  spline S290 degree 3 poles (-41.313, -273.4114) (-41.6067, -274.0004) (-41.9178, -274.6072) (-42.2473, -275.2312) knots 0 0 0 0 1 1 1 1
  spline S291 degree 3 poles (13.9559, -284.6582) (12.8615, -282.3543) (11.94, -280.2066) (11.1655, -278.2308) knots 0 0 0 0 1 1 1 1
  arc A289 (-5.0688, -276.4685) -> (-5.4437, -276.1847) centre (-5.4516, -276.5847) ccw
  arc A290 (-114.9274, -251.1958) -> (-115.3883, -251.2888) centre (-115.0938, -251.5595) ccw
  spline S292 degree 3 poles (130.7796, -245.8327) (130.2625, -245.3526) (129.7685, -244.8826) (129.2967, -244.4236) knots 0 0 0 0 1 1 1 1
  arc A291 (129.2967, -244.4236) -> (128.8313, -244.3566) centre (129.0178, -244.7104) ccw
  spline S293 degree 3 poles (124.5221, -246.8902) (124.6234, -247.5406) (124.7208, -248.2155) (124.8131, -248.9151) knots 0 0 0 0 1 1 1 1
  spline S294 degree 3 poles (-110.9347, -262.5234) (-110.9211, -259.9728) (-110.8195, -257.638) (-110.66, -255.5218) knots 0 0 0 0 1 1 1 1
  spline S295 degree 3 poles (-102.4328, -258.9296) (-103.8164, -260.5388) (-105.3955, -262.2616) (-107.1894, -264.0748) knots 0 0 0 0 1 1 1 1
  spline S296 degree 3 poles (149.9091, -242.3888) (147.8368, -240.9017) (145.9914, -239.4677) (144.3578, -238.1131) knots 0 0 0 0 1 1 1 1
  spline S297 degree 3 poles (116.7899, -252.7789) (116.3006, -252.2705) (115.8336, -251.7735) (115.3883, -251.2888) knots 0 0 0 0 1 1 1 1
  arc A292 (115.3883, -251.2888) -> (114.9274, -251.1958) centre (115.0938, -251.5595) ccw
  arc A293 (110.7207, -253.0782) -> (114.9274, -251.1958) centre (0, 0) ccw
  spline S298 degree 3 poles (107.1894, -264.0748) (105.3955, -262.2616) (103.8164, -260.5388) (102.4328, -258.9296) knots 0 0 0 0 1 1 1 1
  arc A294 (124.7367, -246.4719) -> (128.8313, -244.3566) centre (0, 0) ccw
  arc A295 (121.8275, -257.6492) -> (125.48, -255.8902) centre (0, 0) ccw
  spline S299 degree 3 poles (-124.8131, -248.9151) (-124.7208, -248.2155) (-124.6234, -247.5406) (-124.5221, -246.8902) knots 0 0 0 0 1 1 1 1
  arc A296 (-110.9347, -262.5234) -> (-107.1894, -264.0748) centre (0, 0) ccw
  spline S300 degree 3 poles (110.66, -255.5218) (110.8195, -257.638) (110.9211, -259.9728) (110.9347, -262.5234) knots 0 0 0 0 1 1 1 1
  spline S301 degree 3 poles (-110.66, -255.5218) (-110.607, -254.8182) (-110.5476, -254.1389) (-110.4829, -253.4839) knots 0 0 0 0 1 1 1 1
  arc A297 (96.3563, -258.8882) -> (100.662, -257.2447) centre (0, 0) ccw
  arc A298 (107.1894, -264.0748) -> (110.9347, -262.5234) centre (0, 0) ccw
  arc A299 (-110.4829, -253.4839) -> (-110.7207, -253.0782) centre (-110.881, -253.4447) ccw
  arc A300 (142.7982, -236.7894) -> (142.3298, -236.7485) centre (142.5359, -237.0914) ccw
  spline S302 degree 3 poles (136.0824, -250.4129) (134.0968, -248.812) (132.3347, -247.2768) (130.7796, -245.8327) knots 0 0 0 0 1 1 1 1
  arc A301 (96.3563, -258.8882) -> (96.0962, -259.2799) centre (96.4958, -259.2631) ccw
  arc A302 (-125.48, -255.8902) -> (-121.8275, -257.6492) centre (0, 0) ccw
  spline S303 degree 3 poles (121.8275, -257.6492) (119.9348, -255.9395) (118.2616, -254.3079) (116.7899, -252.7789) knots 0 0 0 0 1 1 1 1
  spline S304 degree 3 poles (110.4829, -253.4839) (110.5476, -254.1389) (110.607, -254.8182) (110.66, -255.5218) knots 0 0 0 0 1 1 1 1
  spline S305 degree 3 poles (96.0962, -259.2799) (96.124, -259.9375) (96.1452, -260.6191) (96.1587, -261.3246) knots 0 0 0 0 1 1 1 1
  spline S306 degree 3 poles (102.4328, -258.9296) (101.9727, -258.3946) (101.5344, -257.8723) (101.1169, -257.3634) knots 0 0 0 0 1 1 1 1
  spline S307 degree 3 poles (96.1587, -261.3246) (96.1992, -263.4464) (96.1698, -265.7832) (96.0404, -268.3306) knots 0 0 0 0 1 1 1 1
  arc A303 (101.1169, -257.3634) -> (100.662, -257.2447) centre (100.8077, -257.6171) ccw
  spline S308 degree 3 poles (92.214, -269.6695) (90.5246, -267.7586) (89.0445, -265.9499) (87.7533, -264.2658) knots 0 0 0 0 1 1 1 1
  arc A304 (92.214, -269.6695) -> (96.0404, -268.3306) centre (0, 0) ccw
  arc A305 (110.7207, -253.0782) -> (110.4829, -253.4839) centre (110.881, -253.4447) ccw
  spline S309 degree 3 poles (124.8131, -248.9151) (125.091, -251.019) (125.3234, -253.3445) (125.48, -255.8902) knots 0 0 0 0 1 1 1 1
  spline S310 degree 3 poles (-116.7899, -252.7789) (-118.2616, -254.3079) (-119.9348, -255.9395) (-121.8275, -257.6492) knots 0 0 0 0 1 1 1 1
  arc A306 (138.3603, -239.0901) -> (138.1694, -239.5198) centre (138.5606, -239.4363) ccw
  arc A307 (138.3603, -239.0901) -> (142.3298, -236.7485) centre (0, 0) ccw
  arc A308 (-96.0962, -259.2799) -> (-96.3563, -258.8882) centre (-96.4958, -259.2631) ccw
  arc A309 (-100.662, -257.2447) -> (-101.1169, -257.3634) centre (-100.8077, -257.6171) ccw
  arc A310 (-114.9274, -251.1958) -> (-110.7207, -253.0782) centre (0, 0) ccw
  arc A311 (-128.8313, -244.3566) -> (-124.7367, -246.4719) centre (0, 0) ccw
  spline S311 degree 3 poles (-125.48, -255.8902) (-125.3234, -253.3445) (-125.091, -251.019) (-124.8131, -248.9151) knots 0 0 0 0 1 1 1 1
  arc A312 (-128.8313, -244.3566) -> (-129.2967, -244.4236) centre (-129.0178, -244.7104) ccw
  arc A313 (-124.5221, -246.8902) -> (-124.7367, -246.4719) centre (-124.9173, -246.8288) ccw
  spline S312 degree 3 poles (144.3578, -238.1131) (143.8146, -237.6627) (143.295, -237.2212) (142.7982, -236.7894) knots 0 0 0 0 1 1 1 1
  spline S313 degree 3 poles (138.1694, -239.5198) (138.307, -240.1635) (138.4421, -240.8319) (138.5736, -241.5251) knots 0 0 0 0 1 1 1 1
  arc A314 (136.0824, -250.4129) -> (139.6305, -248.452) centre (0, 0) ccw
  spline S314 degree 3 poles (138.5736, -241.5251) (138.969, -243.6102) (139.3314, -245.919) (139.6305, -248.452) knots 0 0 0 0 1 1 1 1
  spline S315 degree 3 poles (-115.3883, -251.2888) (-115.8336, -251.7735) (-116.3006, -252.2705) (-116.7899, -252.7789) knots 0 0 0 0 1 1 1 1
  arc A315 (124.7367, -246.4719) -> (124.5221, -246.8902) centre (124.9173, -246.8288) ccw
  arc A316 (76.9484, -274.4157) -> (80.8439, -273.2935) centre (0, 0) ccw
  spline S316 degree 3 poles (275.2977, -25.9177) (275.9023, -26.1779) (276.5255, -26.4545) (277.167, -26.7485) knots 0 0 0 0 1 1 1 1
  arc A317 (270.4716, -56.1496) -> (270.6648, -56.5783) centre (270.8632, -56.2309) ccw
  arc A318 (81.6887, -263.8837) -> (86.0798, -262.4841) centre (0, 0) ccw
  arc A319 (66.7641, -268.0489) -> (71.2268, -266.8977) centre (0, 0) ccw
  spline S317 degree 3 poles (273.4114, -41.313) (274.0004, -41.6067) (274.6072, -41.9178) (275.2312, -42.2473) knots 0 0 0 0 1 1 1 1
  arc A320 (273.1944, -40.8958) -> (273.8386, -36.3324) centre (0, 0) ccw
  spline S318 degree 3 poles (270.4478, -66.295) (269.7452, -66.3606) (269.0656, -66.4158) (268.409, -66.4618) knots 0 0 0 0 1 1 1 1
  arc A321 (274.1626, -35.9916) -> (273.8386, -36.3324) centre (274.2352, -36.385) ccw
  spline S319 degree 3 poles (277.167, -26.7485) (279.0963, -27.6326) (281.1889, -28.673) (283.4279, -29.8949) knots 0 0 0 0 1 1 1 1
  arc A322 (271.7132, -51.3074) -> (271.3707, -51.6295) centre (271.7636, -51.7042) ccw
  arc A323 (276.4685, -5.0688) -> (276.1847, -5.4437) centre (276.5847, -5.4516) ccw
  spline S320 degree 3 poles (284.9929, -2.027) (282.6312, -2.9904) (280.4352, -3.79) (278.4191, -4.4526) knots 0 0 0 0 1 1 1 1
  arc A324 (275.7494, -20.5626) -> (275.445, -20.921) centre (275.8439, -20.9513) ccw
  spline S321 degree 3 poles (284.4309, -18.0035) (282.0189, -18.833) (279.7816, -19.5082) (277.7315, -20.0566) knots 0 0 0 0 1 1 1 1
  spline S322 degree 3 poles (270.6648, -56.5783) (271.2365, -56.9046) (271.8248, -57.2492) (272.4294, -57.6132) knots 0 0 0 0 1 1 1 1
  arc A325 (277.3965, -65.393) -> (278.2986, -61.4407) centre (0, 0) ccw
  arc A326 (284.9929, -2.027) -> (284.9929, 2.027) centre (0, 0) ccw
  arc A327 (275.0576, -25.5134) -> (275.445, -20.921) centre (0, 0) ccw
  arc A328 (270.4716, -56.1496) -> (271.3707, -51.6295) centre (0, 0) ccw
  spline S323 degree 3 poles (282.974, -33.9233) (280.5193, -34.6163) (278.2476, -35.165) (276.1699, -35.5976) knots 0 0 0 0 1 1 1 1
  spline S324 degree 3 poles (267.0666, -71.6656) (267.6191, -72.0234) (268.1872, -72.4005) (268.7704, -72.7978) knots 0 0 0 0 1 1 1 1
  arc A329 (266.8977, -71.2268) -> (267.0666, -71.6656) centre (267.2842, -71.3299) ccw
  spline S325 degree 3 poles (81.407, -264.2602) (81.398, -264.9183) (81.381, -265.6) (81.3548, -266.3051) knots 0 0 0 0 1 1 1 1
  arc A330 (81.6887, -263.8837) -> (81.407, -264.2602) centre (81.807, -264.2658) ccw
  arc A331 (66.7641, -268.0489) -> (66.4618, -268.409) centre (66.8608, -268.437) ccw
  spline S326 degree 3 poles (278.4191, 4.4526) (280.4352, 3.79) (282.6312, 2.9904) (284.9929, 2.027) knots 0 0 0 0 1 1 1 1
  spline S327 degree 3 poles (76.9484, -274.4157) (75.3688, -272.4131) (73.9925, -270.5243) (72.7978, -268.7704) knots 0 0 0 0 1 1 1 1
  spline S328 degree 3 poles (72.7978, -268.7704) (72.4005, -268.1872) (72.0234, -267.6191) (71.6656, -267.0666) knots 0 0 0 0 1 1 1 1
  spline S329 degree 3 poles (276.4685, 5.0688) (277.0984, 4.8779) (277.7488, 4.6729) (278.4191, 4.4526) knots 0 0 0 0 1 1 1 1
  arc A332 (275.0576, -25.5134) -> (275.2977, -25.9177) centre (275.4559, -25.5503) ccw
  spline S330 degree 3 poles (273.7395, -51.0266) (273.0417, -51.1315) (272.3662, -51.2247) (271.7132, -51.3074) knots 0 0 0 0 1 1 1 1
  arc A333 (268.409, -66.4618) -> (268.0489, -66.7641) centre (268.437, -66.8608) ccw
  arc A334 (266.8977, -71.2268) -> (268.0489, -66.7641) centre (0, 0) ccw
  spline S331 degree 3 poles (268.7704, -72.7978) (270.5243, -73.9925) (272.4131, -75.3688) (274.4157, -76.9484) knots 0 0 0 0 1 1 1 1
  spline S332 degree 3 poles (278.4191, -4.4526) (277.7488, -4.6729) (277.0984, -4.8779) (276.4685, -5.0688) knots 0 0 0 0 1 1 1 1
  spline S333 degree 3 poles (66.295, -270.4478) (66.0977, -272.5608) (65.8068, -274.8797) (65.393, -277.3965) knots 0 0 0 0 1 1 1 1
  spline S334 degree 3 poles (277.7315, -20.0566) (277.0498, -20.239) (276.389, -20.4073) (275.7494, -20.5626) knots 0 0 0 0 1 1 1 1
  spline S335 degree 3 poles (87.7533, -264.2658) (87.324, -263.7058) (86.9156, -263.1597) (86.5274, -262.6282) knots 0 0 0 0 1 1 1 1
  arc A335 (284.4309, -18.0035) -> (284.6582, -13.9559) centre (0, 0) ccw
  arc A336 (86.5274, -262.6282) -> (86.0798, -262.4841) centre (86.2044, -262.8642) ccw
  spline S336 degree 3 poles (66.4618, -268.409) (66.4158, -269.0656) (66.3606, -269.7452) (66.295, -270.4478) knots 0 0 0 0 1 1 1 1
  spline S337 degree 3 poles (81.3548, -266.3051) (81.2764, -268.4259) (81.1159, -270.7574) (80.8439, -273.2935) knots 0 0 0 0 1 1 1 1
  arc A337 (61.4407, -278.2986) -> (65.393, -277.3965) centre (0, 0) ccw